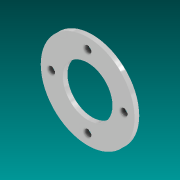
# Autodesk Inventor part: 60mmspacer
Saved by Autodesk Inventor 2020.3 (Build 243373000, 373)
## iProperties
Created: 2020-05-23
Part Number: 60mmspacer
Material: Aluminum 6061
Document SubType Name: Sheet Metal
Designer: Svend
Density: 2.7 g/cm^3
Sheet Metal Rule: Default_mm
Appearance: Aluminum - Polished
Author: Svend
Autodesk Inventor part; units mm, degrees
ref_plane "YZ Plane" through (0, 0, 0) normal (1, 0, 0) x (0, 1, 0)
ref_plane "XZ Plane" through (0, 0, 0) normal (0, 1, 0) x (-1, 0, 0)
ref_plane "XY Plane" through (0, 0, 0) normal (0, 0, 1) x (1, 0, 0)
sketch "Sketch1" plane through (0, 0, 0) normal (0, 0, 1) x (1, 0, 0)
  circle A0 centre (0, 0) radius 11
  circle A1 centre (0, 0) radius 20.6625
  point P0 (16, 0)
  point P1 (0, 16)
  point P2 (-16, 0)
  point P3 (0, -16)
  dimension "d0" = 22
  dimension "d2" = 16
  dimension "d5" = 360
  dimension "d7" = 41.325
  constraints: 2 centre point, 2 coincident, 1 horizontal alignment, 5 other
  measures "d0" diameter of A0
  measures "d2" distance of A0.centre point (16, 0)
  measures "d7" diameter of A1
extrude "Plate1" add sketch "Sketch1" along normal blind 2
hole "Hole1" at (16, 0, 0) at (0, 16, 0) at (-16, 0, 0) at (0, -16, 0) direction (0, 0, 1) diameter 3.2 end through all clearance for "Countersunk Flat Head Screw ISO 2009/7046" size "M3" standard "ISO"
equation "\"d14\" = Thickness"
equation "\"d8\" = Thickness"
equation "\"BendRadius\" = Thickness"
equation "\"BendReliefWidth\" = Thickness"
equation "\"BendReliefDepth\" = 0.5 * Thickness"
equation "\"CornerReliefSize\" = 4 * Thickness"
equation "\"MinimumRemnant\" = 2 * Thickness"
equation "\"TransitionRadius\" = BendRadius"
equation "\"JacobiRadiusSize\" = BendRadius"
equation "\"GapSize\" = Thickness"
equation "\"Thickness\" = 2"
body "Solid1"
